Autodesk Fusion 360 part; units mm, degrees
(part 11 of 14)
  line L5327 (75.3115, 39.124) -> (75.7865, 39.124)
  line L5328 (77.3, 16.876) -> (76.5, 16.876)
  line L5329 (74.549, 38.8615) -> (74.549, 38.3865)
  line L5330 (75.3115, 40.124) -> (75.7865, 40.124)
  arc A2944 (81.0876, 38.2211) -> (81.0876, 38.4521) centre (81.0876, 38.3366) ccw
  line L5331 (75.049, 38.8615) -> (75.049, 38.3865)
  line L5332 (73.3115, 40.124) -> (73.7865, 40.124)
  arc A2945 (75.549, 38.6748) -> (75.549, 38.5732) centre (75.549, 38.624) ccw
  line L5333 (75.049, 40.8615) -> (75.049, 40.3865)
  line L5334 (75.3115, 39.624) -> (75.7865, 39.624)
  line L5335 (75.049, 38.8615) -> (75.049, 38.3865)
  arc A2946 (83.042, 40.8018) -> (83.042, 40.7002) centre (83.042, 40.751) ccw
  line L5336 (80.091, 16.622) -> (79.291, 16.622)
  line L5337 (73.3115, 39.124) -> (73.7865, 39.124)
  arc A2947 (75.549, 38.5732) -> (75.549, 38.6748) centre (75.549, 38.624) ccw
  line L5338 (75.549, 40.624) -> (73.549, 40.624)
  line L5339 (74.549, 40.174) -> (74.549, 39.074)
  line L5340 (74.049, 38.8615) -> (74.049, 38.3865)
  line L5341 (75.3115, 39.624) -> (75.7865, 39.624)
  line L5342 (74.549, 40.174) -> (74.549, 39.074)
  line L5343 (80.091, 17.272) -> (79.291, 17.272)
  line L5344 (73.549, 40.624) -> (73.549, 38.624)
  line L5345 (77.3, 16.876) -> (76.5, 16.876)
  line L5346 (80.091, 16.622) -> (79.291, 16.622)
  arc A2948 (75.5034, 40.9229) -> (75.5034, 41.1539) centre (75.5034, 41.0384) ccw
  line L5347 (74.049, 38.8615) -> (74.049, 38.3865)
  line L5348 (74.549, 40.8615) -> (74.549, 40.3865)
  line L5349 (73.3115, 40.124) -> (73.7865, 40.124)
  line L5350 (74.549, 40.174) -> (74.549, 39.074)
  line L5351 (75.049, 40.8615) -> (75.049, 40.3865)
  arc A2949 (75.549, 40.6748) -> (75.549, 40.5732) centre (75.549, 40.624) ccw
  line L5352 (74.049, 40.8615) -> (74.049, 40.3865)
  line L5353 (75.9, 17.526) -> (75.1, 17.526)
  line L5354 (74.549, 40.8615) -> (74.549, 40.3865)
  arc A2950 (73.549, 38.6748) -> (73.549, 38.5732) centre (73.549, 38.624) ccw
  line L5355 (75.9, 18.176) -> (75.1, 18.176)
  arc A2951 (77.559, 16.5214) -> (77.559, 16.1966) centre (77.559, 16.359) ccw
  arc A2952 (73.549, 40.5732) -> (73.549, 40.6748) centre (73.549, 40.624) ccw
  arc A2953 (73.549, 38.5732) -> (73.549, 38.6748) centre (73.549, 38.624) ccw
  line L5356 (74.549, 40.8615) -> (74.549, 40.3865)
  line L5357 (73.3115, 39.624) -> (73.7865, 39.624)
  line L5358 (73.3115, 39.624) -> (73.7865, 39.624)
  line L5359 (75.549, 38.624) -> (75.549, 40.624)
  line L5360 (74.049, 40.8615) -> (74.049, 40.3865)
  line L5361 (73.3115, 40.124) -> (73.7865, 40.124)
  line L5362 (73.3115, 39.124) -> (73.7865, 39.124)
  line L5363 (73.549, 38.624) -> (75.549, 38.624)
  line L5364 (75.3115, 39.124) -> (75.7865, 39.124)
  line L5365 (75.9, 16.876) -> (75.1, 16.876)
  line L5366 (73.3115, 39.624) -> (73.7865, 39.624)
  arc A2954 (75.549, 40.5732) -> (75.549, 40.6748) centre (75.549, 40.624) ccw
  line L5367 (75.3115, 39.124) -> (75.7865, 39.124)
  line L5368 (74.549, 38.8615) -> (74.549, 38.3865)
  line L5369 (74.049, 38.8615) -> (74.049, 38.3865)
  line L5370 (75.9, 16.876) -> (75.1, 16.876)
  line L5371 (75.049, 40.8615) -> (75.049, 40.3865)
  arc A2955 (9.1123, 16.129) -> (11.2078, 16.129) centre (10.16, 16.129) ccw
  arc A2956 (10.16, 16.9227) -> (10.16, 15.3352) centre (10.16, 16.129) ccw
  arc A2957 (12.2555, 16.129) -> (8.0645, 16.129) centre (10.16, 16.129) ccw
  arc A2958 (10.16, 15.3352) -> (10.16, 16.9227) centre (10.16, 16.129) ccw
  arc A2959 (7.8105, 16.129) -> (12.5095, 16.129) centre (10.16, 16.129) ccw
  line L5372 (8.6783, 17.6107) -> (8.4987, 17.7903)
  line L5373 (11.507, 17.476) -> (11.8213, 17.7903)
  arc A2960 (9.2075, 16.129) -> (11.1125, 16.129) centre (10.16, 16.129) ccw
  line L5374 (11.6417, 17.6107) -> (11.8213, 17.7903)
  line L5375 (10.414, 16.129) -> (9.906, 16.129)
  line L5376 (10.414, 16.129) -> (9.906, 16.129)
  arc A2961 (10.16, 16.9227) -> (10.16, 15.3352) centre (10.16, 16.129) ccw
  arc A2962 (10.16, 16.9227) -> (10.16, 15.3352) centre (10.16, 16.129) ccw
  arc A2963 (12.5095, 16.129) -> (7.8105, 16.129) centre (10.16, 16.129) ccw
  arc A2964 (11.1125, 16.129) -> (9.2075, 16.129) centre (10.16, 16.129) ccw
  line L5377 (8.6783, 17.6107) -> (8.4987, 17.7903)
  line L5378 (11.6417, 14.6473) -> (11.8213, 14.4677)
  line L5379 (11.6417, 14.6473) -> (11.8213, 14.4677)
  arc A2965 (10.16, 16.9227) -> (10.16, 15.3352) centre (10.16, 16.129) ccw
  line L5380 (10.16, 15.875) -> (10.16, 16.383)
  line L5381 (10.16, 15.875) -> (10.16, 16.383)
  line L5382 (6.35, 11.43) -> (6.35, 11.938)
  arc A2966 (11.2078, 16.129) -> (9.1123, 16.129) centre (10.16, 16.129) ccw
  line L5383 (6.35, 11.43) -> (6.35, 11.938)
  line L5384 (6.35, 11.43) -> (6.35, 11.938)
  line L5385 (6.604, 11.684) -> (6.096, 11.684)
  arc A2967 (10.16, 16.9227) -> (10.16, 15.3352) centre (10.16, 16.129) ccw
  line L5386 (11.6417, 17.6107) -> (11.8213, 17.7903)
  arc A2968 (8.0645, 16.129) -> (12.2555, 16.129) centre (10.16, 16.129) ccw
  arc A2969 (10.16, 15.3352) -> (10.16, 16.9227) centre (10.16, 16.129) ccw
  line L5387 (5.6061, 17.9251) -> (5.6959, 18.0149)
  line L5388 (10.414, 16.129) -> (9.906, 16.129)
  arc A2970 (8.0645, 16.129) -> (12.2555, 16.129) centre (10.16, 16.129) ccw
  arc A2971 (12.5095, 16.129) -> (7.8105, 16.129) centre (10.16, 16.129) ccw
  line L5389 (10.16, 15.875) -> (10.16, 16.383)
  arc A2972 (10.16, 15.3352) -> (10.16, 16.9227) centre (10.16, 16.129) ccw
  arc A2973 (12.5095, 16.129) -> (7.8105, 16.129) centre (10.16, 16.129) ccw
  arc A2974 (10.16, 16.9227) -> (10.16, 15.3352) centre (10.16, 16.129) ccw
  line L5390 (10.414, 16.129) -> (9.906, 16.129)
  line L5391 (10.414, 16.129) -> (9.906, 16.129)
  line L5392 (10.16, 15.875) -> (10.16, 16.383)
  arc A2975 (12.065, 16.129) -> (8.255, 16.129) centre (10.16, 16.129) ccw
  line L5393 (10.414, 16.129) -> (9.906, 16.129)
  line L5394 (11.507, 14.782) -> (11.8213, 14.4677)
  line L5395 (10.414, 16.129) -> (9.906, 16.129)
  arc A2976 (7.8105, 16.129) -> (12.5095, 16.129) centre (10.16, 16.129) ccw
  arc A2977 (12.2555, 16.129) -> (8.0645, 16.129) centre (10.16, 16.129) ccw
  line L5396 (10.16, 15.875) -> (10.16, 16.383)
  arc A2978 (10.16, 15.3352) -> (10.16, 16.9227) centre (10.16, 16.129) ccw
  arc A2979 (10.16, 15.3352) -> (10.16, 16.9227) centre (10.16, 16.129) ccw
  arc A2980 (9.1123, 16.129) -> (11.2078, 16.129) centre (10.16, 16.129) ccw
  line L5397 (10.16, 15.875) -> (10.16, 16.383)
  line L5398 (8.6783, 14.6473) -> (8.4987, 14.4677)
  arc A2981 (7.8105, 16.129) -> (12.5095, 16.129) centre (10.16, 16.129) ccw
  arc A2982 (10.16, 15.3352) -> (10.16, 16.9227) centre (10.16, 16.129) ccw
  line L5399 (10.16, 15.875) -> (10.16, 16.383)
  line L5400 (8.813, 14.782) -> (8.4987, 14.4677)
  line L5401 (10.16, 15.875) -> (10.16, 16.383)
  line L5402 (8.6783, 14.6473) -> (8.4987, 14.4677)
  arc A2983 (10.16, 16.9227) -> (10.16, 15.3352) centre (10.16, 16.129) ccw
  arc A2984 (11.2078, 16.129) -> (9.1123, 16.129) centre (10.16, 16.129) ccw
  line L5403 (8.813, 17.476) -> (8.4987, 17.7903)
  arc A2985 (8.255, 16.129) -> (12.065, 16.129) centre (10.16, 16.129) ccw
  arc A2986 (10.16, 15.3352) -> (10.16, 16.9227) centre (10.16, 16.129) ccw
  arc A2987 (8.255, 11.684) -> (4.445, 11.684) centre (6.35, 11.684) ccw
  line L5404 (63.5, 5.588) -> (64.77, 6.858)
  line L5405 (60.96, 5.588) -> (62.23, 5.588)
  line L5406 (62.23, 6.858) -> (60.96, 6.858)
  line L5407 (59.69, 6.858) -> (58.42, 6.858)
  arc A2988 (6.35, 10.8902) -> (6.35, 12.4777) centre (6.35, 11.684) ccw
  arc A2989 (6.35, 10.8902) -> (6.35, 12.4777) centre (6.35, 11.684) ccw
  arc A2990 (11.2078, 16.129) -> (9.1123, 16.129) centre (10.16, 16.129) ccw
  line L5408 (6.35, 11.43) -> (6.35, 11.938)
  arc A2991 (4.2545, 11.684) -> (8.4455, 11.684) centre (6.35, 11.684) ccw
  arc A2992 (6.35, 12.4777) -> (6.35, 10.8902) centre (6.35, 11.684) ccw
  line L5409 (5.003, 13.031) -> (4.6887, 13.3453)
  arc A2993 (6.35, 10.8902) -> (6.35, 12.4777) centre (6.35, 11.684) ccw
  arc A2994 (4.0005, 11.684) -> (8.6995, 11.684) centre (6.35, 11.684) ccw
  arc A2995 (7.3978, 11.684) -> (5.3023, 11.684) centre (6.35, 11.684) ccw
  arc A2996 (6.35, 10.8902) -> (6.35, 12.4777) centre (6.35, 11.684) ccw
  line L5410 (6.35, 11.43) -> (6.35, 11.938)
  arc A2997 (6.35, 12.4777) -> (6.35, 10.8902) centre (6.35, 11.684) ccw
  arc A2998 (6.35, 12.4777) -> (6.35, 10.8902) centre (6.35, 11.684) ccw
  line L5411 (4.8683, 10.2023) -> (4.6887, 10.0227)
  line L5412 (57.15, 5.588) -> (55.88, 6.858)
  arc A2999 (6.35, 10.8902) -> (6.35, 12.4777) centre (6.35, 11.684) ccw
  arc A3000 (11.2078, 16.129) -> (9.1123, 16.129) centre (10.16, 16.129) ccw
  line L5413 (6.604, 11.684) -> (6.096, 11.684)
  arc A3001 (9.1123, 16.129) -> (11.2078, 16.129) centre (10.16, 16.129) ccw
  line L5414 (53.34, 5.588) -> (54.61, 6.858)
  line L5415 (7.8317, 13.1657) -> (8.0113, 13.3453)
  line L5416 (64.77, 5.588) -> (64.77, 6.858)
  arc A3002 (6.35, 10.8902) -> (6.35, 12.4777) centre (6.35, 11.684) ccw
  line L5417 (62.23, 5.588) -> (62.23, 6.858)
  line L5418 (7.8317, 10.2023) -> (8.0113, 10.0227)
  line L5419 (6.35, 11.43) -> (6.35, 11.938)
  line L5420 (55.88, 5.588) -> (57.15, 6.858)
  arc A3003 (5.3023, 11.684) -> (7.3978, 11.684) centre (6.35, 11.684) ccw
  line L5421 (52.705, 7.493) -> (52.705, 2.413)
  arc A3004 (6.35, 12.4777) -> (6.35, 10.8902) centre (6.35, 11.684) ccw
  line L5422 (6.604, 11.684) -> (6.096, 11.684)
  line L5423 (6.35, 11.43) -> (6.35, 11.938)
  arc A3005 (5.3023, 11.684) -> (7.3978, 11.684) centre (6.35, 11.684) ccw
  arc A3006 (6.35, 12.4777) -> (6.35, 10.8902) centre (6.35, 11.684) ccw
  arc A3007 (6.35, 10.8902) -> (6.35, 12.4777) centre (6.35, 11.684) ccw
  arc A3008 (6.35, 12.4777) -> (6.35, 10.8902) centre (6.35, 11.684) ccw
  arc A3009 (6.35, 12.4777) -> (6.35, 10.8902) centre (6.35, 11.684) ccw
  line L5424 (6.35, 11.43) -> (6.35, 11.938)
  line L5425 (6.604, 11.684) -> (6.096, 11.684)
  line L5426 (6.604, 11.684) -> (6.096, 11.684)
  line L5427 (6.604, 11.684) -> (6.096, 11.684)
  line L5428 (6.35, 11.43) -> (6.35, 11.938)
  line L5429 (6.604, 11.684) -> (6.096, 11.684)
  line L5430 (6.604, 11.684) -> (6.096, 11.684)
  arc A3010 (6.35, 12.4777) -> (6.35, 10.8902) centre (6.35, 11.684) ccw
  line L5431 (6.604, 11.684) -> (6.096, 11.684)
  line L5432 (6.604, 11.684) -> (6.096, 11.684)
  line L5433 (6.35, 11.43) -> (6.35, 11.938)
  arc A3011 (6.35, 10.8902) -> (6.35, 12.4777) centre (6.35, 11.684) ccw
  arc A3012 (6.35, 12.4777) -> (6.35, 10.8902) centre (6.35, 11.684) ccw
  arc A3013 (6.35, 10.8902) -> (6.35, 12.4777) centre (6.35, 11.684) ccw
  arc A3014 (6.35, 12.4777) -> (6.35, 10.8902) centre (6.35, 11.684) ccw
  arc A3015 (8.4455, 11.684) -> (4.2545, 11.684) centre (6.35, 11.684) ccw
  arc A3016 (4.2545, 11.684) -> (8.4455, 11.684) centre (6.35, 11.684) ccw
  line L5434 (7.8317, 10.2023) -> (8.0113, 10.0227)
  arc A3017 (9.1123, 16.129) -> (11.2078, 16.129) centre (10.16, 16.129) ccw
  line L5435 (4.8683, 13.1657) -> (4.6887, 13.3453)
  arc A3018 (6.35, 10.8902) -> (6.35, 12.4777) centre (6.35, 11.684) ccw
  line L5436 (54.61, 5.588) -> (54.61, 6.858)
  line L5437 (65.405, 7.493) -> (52.705, 7.493)
  arc A3019 (5.3023, 11.684) -> (7.3978, 11.684) centre (6.35, 11.684) ccw
  line L5438 (4.8683, 13.1657) -> (4.6887, 13.3453)
  line L5439 (64.77, 6.858) -> (63.5, 6.858)
  line L5440 (55.88, 6.858) -> (55.88, 5.588)
  line L5441 (58.42, 3.048) -> (59.69, 3.048)
  line L5442 (60.96, 6.858) -> (60.96, 5.588)
  arc A3020 (8.4455, 11.684) -> (4.2545, 11.684) centre (6.35, 11.684) ccw
  line L5443 (64.77, 3.048) -> (64.77, 4.318)
  line L5444 (58.42, 4.318) -> (58.42, 3.048)
  arc A3021 (4.0005, 11.684) -> (8.6995, 11.684) centre (6.35, 11.684) ccw
  line L5445 (58.42, 5.588) -> (59.69, 6.858)
  arc A3022 (8.6995, 11.684) -> (4.0005, 11.684) centre (6.35, 11.684) ccw
  arc A3023 (7.3025, 11.684) -> (5.3975, 11.684) centre (6.35, 11.684) ccw
  line L5446 (63.5, 6.858) -> (63.5, 5.588)
  line L5447 (55.88, 3.048) -> (57.15, 3.048)
  line L5448 (53.975, 3.937) -> (53.975, 3.429)
  line L5449 (60.325, 2.413) -> (60.325, 7.493)
  line L5450 (57.15, 6.858) -> (55.88, 6.858)
  line L5451 (52.705, 2.413) -> (65.405, 2.413)
  line L5452 (55.88, 5.588) -> (57.15, 5.588)
  line L5453 (52.705, 7.493) -> (52.705, 2.413)
  line L5454 (64.77, 4.318) -> (63.5, 4.318)
  line L5455 (60.96, 4.318) -> (60.96, 3.048)
  line L5456 (57.15, 4.318) -> (55.88, 4.318)
  line L5457 (7.697, 10.337) -> (8.0113, 10.0227)
  line L5458 (58.42, 3.048) -> (59.69, 4.318)
  line L5459 (59.69, 3.048) -> (59.69, 4.318)
  line L5460 (62.23, 5.588) -> (60.96, 6.858)
  arc A3024 (5.3975, 11.684) -> (7.3025, 11.684) centre (6.35, 11.684) ccw
  arc A3025 (7.3978, 11.684) -> (5.3023, 11.684) centre (6.35, 11.684) ccw
  line L5461 (59.69, 5.588) -> (58.42, 6.858)
  line L5462 (60.96, 5.588) -> (62.23, 6.858)
  line L5463 (5.003, 10.337) -> (4.6887, 10.0227)
  line L5464 (54.61, 4.318) -> (53.34, 4.318)
  line L5465 (58.42, 6.858) -> (58.42, 5.588)
  arc A3026 (7.3978, 11.684) -> (5.3023, 11.684) centre (6.35, 11.684) ccw
  arc A3027 (8.6995, 11.684) -> (4.0005, 11.684) centre (6.35, 11.684) ccw
  line L5466 (7.697, 13.031) -> (8.0113, 13.3453)
  arc A3028 (5.3023, 11.684) -> (7.3978, 11.684) centre (6.35, 11.684) ccw
  line L5467 (62.23, 3.048) -> (62.23, 4.318)
  line L5468 (59.69, 5.588) -> (59.69, 6.858)
  line L5469 (63.5, 5.588) -> (64.77, 5.588)
  line L5470 (59.69, 3.048) -> (58.42, 4.318)
  line L5471 (62.23, 3.048) -> (60.96, 4.318)
  line L5472 (60.96, 3.048) -> (62.23, 4.318)
  line L5473 (53.34, 5.588) -> (54.61, 5.588)
  line L5474 (57.785, 2.413) -> (57.785, 7.493)
  line L5475 (54.61, 5.588) -> (53.34, 6.858)
  line L5476 (65.405, 7.493) -> (52.705, 7.493)
  arc A3029 (7.3978, 11.684) -> (5.3023, 11.684) centre (6.35, 11.684) ccw
  line L5477 (62.865, 2.413) -> (62.865, 7.493)
  line L5478 (53.34, 3.048) -> (54.61, 3.048)
  line L5479 (64.77, 5.588) -> (63.5, 6.858)
  line L5480 (65.405, 2.413) -> (65.405, 7.493)
  arc A3030 (54.2227, 3.683) -> (53.7274, 3.683) centre (53.975, 3.683) ccw
  arc A3031 (4.445, 11.684) -> (8.255, 11.684) centre (6.35, 11.684) ccw
  line L5481 (52.705, 2.413) -> (65.405, 2.413)
  line L5482 (55.88, 3.048) -> (57.15, 4.318)
  line L5483 (54.61, 3.048) -> (53.34, 4.318)
  line L5484 (55.88, 4.318) -> (55.88, 3.048)
  line L5485 (62.23, 4.318) -> (60.96, 4.318)
  line L5486 (57.15, 3.048) -> (55.88, 4.318)
  line L5487 (53.975, 6.477) -> (53.975, 5.969)
  arc A3032 (54.2227, 3.683) -> (53.7274, 3.683) centre (53.975, 3.683) ccw
  line L5488 (54.229, 3.683) -> (53.721, 3.683)
  arc A3033 (53.7274, 3.683) -> (54.2227, 3.683) centre (53.975, 3.683) ccw
  line L5489 (53.975, 3.937) -> (53.975, 3.429)
  line L5490 (63.5, 3.048) -> (64.77, 4.318)
  line L5491 (57.15, 5.588) -> (57.15, 6.858)
  line L5492 (53.34, 3.048) -> (54.61, 4.318)
  line L5493 (54.229, 3.683) -> (53.721, 3.683)
  line L5494 (58.42, 5.588) -> (59.69, 5.588)
  line L5495 (53.975, 6.477) -> (53.975, 5.969)
  line L5496 (54.7624, 3.683) -> (53.1876, 3.683)
  arc A3034 (53.7274, 3.683) -> (54.2227, 3.683) centre (53.975, 3.683) ccw
  line L5497 (54.229, 6.223) -> (53.721, 6.223)
  arc A3035 (53.7274, 3.683) -> (54.2227, 3.683) centre (53.975, 3.683) ccw
  line L5498 (54.7624, 3.683) -> (53.1876, 3.683)
  line L5499 (63.5, 3.048) -> (64.77, 3.048)
  arc A3036 (53.7274, 3.683) -> (54.2227, 3.683) centre (53.975, 3.683) ccw
  line L5500 (54.229, 6.223) -> (53.721, 6.223)
  arc A3037 (54.2227, 3.683) -> (53.7274, 3.683) centre (53.975, 3.683) ccw
  line L5501 (54.61, 3.048) -> (54.61, 4.318)
  line L5502 (57.15, 3.048) -> (57.15, 4.318)
  arc A3038 (53.975, 3.429) -> (53.975, 3.937) centre (53.975, 3.683) ccw
  line L5503 (53.975, 6.477) -> (53.975, 5.969)
  line L5504 (54.229, 3.683) -> (53.721, 3.683)
  line L5505 (53.975, 6.477) -> (53.975, 5.969)
  arc A3039 (53.7274, 3.683) -> (54.2227, 3.683) centre (53.975, 3.683) ccw
  arc A3040 (54.2227, 6.223) -> (53.7274, 6.223) centre (53.975, 6.223) ccw
  line L5506 (64.77, 3.048) -> (63.5, 4.318)
  line L5507 (54.7624, 3.683) -> (53.1876, 3.683)
  line L5508 (53.34, 4.318) -> (53.34, 3.048)
  arc A3041 (54.2227, 3.683) -> (53.7274, 3.683) centre (53.975, 3.683) ccw
  arc A3042 (54.2227, 3.683) -> (53.7274, 3.683) centre (53.975, 3.683) ccw
  arc A3043 (53.7274, 3.683) -> (54.2227, 3.683) centre (53.975, 3.683) ccw
  line L5509 (63.5, 4.318) -> (63.5, 3.048)
  line L5510 (54.229, 3.683) -> (53.721, 3.683)
  arc A3044 (54.2227, 6.223) -> (53.7274, 6.223) centre (53.975, 6.223) ccw
  arc A3045 (53.7274, 3.683) -> (54.2227, 3.683) centre (53.975, 3.683) ccw
  line L5511 (59.69, 4.318) -> (58.42, 4.318)
  line L5512 (54.229, 3.683) -> (53.721, 3.683)
  line L5513 (53.975, 3.937) -> (53.975, 3.429)
  arc A3046 (54.2227, 6.223) -> (53.7274, 6.223) centre (53.975, 6.223) ccw
  line L5514 (54.7624, 3.683) -> (53.1876, 3.683)
  arc A3047 (53.7274, 3.683) -> (54.2227, 3.683) centre (53.975, 3.683) ccw
  line L5515 (54.229, 3.683) -> (53.721, 3.683)
  arc A3048 (53.975, 4.0767) -> (53.975, 3.2893) centre (53.975, 3.683) ccw
  line L5516 (55.245, 2.413) -> (55.245, 7.493)
  line L5517 (53.34, 6.858) -> (53.34, 5.588)
  arc A3049 (53.975, 3.937) -> (53.975, 3.429) centre (53.975, 3.683) ccw
  line L5518 (53.975, 3.937) -> (53.975, 3.429)
  line L5519 (60.96, 3.048) -> (62.23, 3.048)
  line L5520 (65.405, 2.413) -> (65.405, 7.493)
  arc A3050 (54.2227, 3.683) -> (53.7274, 3.683) centre (53.975, 3.683) ccw
  arc A3051 (53.7274, 3.683) -> (54.2227, 3.683) centre (53.975, 3.683) ccw
  line L5521 (54.229, 3.683) -> (53.721, 3.683)
  arc A3052 (54.2227, 3.683) -> (53.7274, 3.683) centre (53.975, 3.683) ccw
  line L5522 (54.61, 6.858) -> (53.34, 6.858)
  line L5523 (53.975, 3.937) -> (53.975, 3.429)
  line L5524 (53.975, 3.937) -> (53.975, 3.429)
  arc A3053 (53.975, 3.2893) -> (53.975, 4.0767) centre (53.975, 3.683) ccw
  line L5525 (54.229, 6.223) -> (53.721, 6.223)
  arc A3054 (53.7274, 6.223) -> (54.2227, 6.223) centre (53.975, 6.223) ccw
  arc A3055 (54.2227, 3.683) -> (53.7274, 3.683) centre (53.975, 3.683) ccw
  line L5526 (54.229, 3.683) -> (53.721, 3.683)
  arc A3056 (56.7627, 3.683) -> (56.2674, 3.683) centre (56.515, 3.683) ccw
  line L5527 (53.975, 6.477) -> (53.975, 5.969)
  line L5528 (53.975, 3.937) -> (53.975, 3.429)
  line L5529 (53.975, 3.937) -> (53.975, 3.429)
  arc A3057 (56.2674, 3.683) -> (56.7627, 3.683) centre (56.515, 3.683) ccw
  arc A3058 (54.2227, 6.223) -> (53.7274, 6.223) centre (53.975, 6.223) ccw
  arc A3059 (56.2674, 3.683) -> (56.7627, 3.683) centre (56.515, 3.683) ccw
  line L5530 (54.229, 6.223) -> (53.721, 6.223)
  line L5531 (53.975, 6.477) -> (53.975, 5.969)
  line L5532 (53.975, 3.937) -> (53.975, 3.429)
  line L5533 (54.229, 6.223) -> (53.721, 6.223)
  arc A3060 (56.2674, 3.683) -> (56.7627, 3.683) centre (56.515, 3.683) ccw
  arc A3061 (56.2674, 3.683) -> (56.7627, 3.683) centre (56.515, 3.683) ccw
  arc A3062 (56.7627, 3.683) -> (56.2674, 3.683) centre (56.515, 3.683) ccw
  arc A3063 (56.2674, 3.683) -> (56.7627, 3.683) centre (56.515, 3.683) ccw
  line L5534 (56.515, 3.937) -> (56.515, 3.429)
  arc A3064 (53.7274, 6.223) -> (54.2227, 6.223) centre (53.975, 6.223) ccw
  arc A3065 (54.2227, 3.683) -> (53.7274, 3.683) centre (53.975, 3.683) ccw
  line L5535 (56.515, 3.937) -> (56.515, 3.429)
  arc A3066 (53.975, 6.477) -> (53.975, 5.969) centre (53.975, 6.223) ccw
  arc A3067 (54.2227, 6.223) -> (53.7274, 6.223) centre (53.975, 6.223) ccw
  arc A3068 (53.7274, 6.223) -> (54.2227, 6.223) centre (53.975, 6.223) ccw
  arc A3069 (54.2227, 6.223) -> (53.7274, 6.223) centre (53.975, 6.223) ccw
  line L5536 (56.515, 3.937) -> (56.515, 3.429)
  line L5537 (56.769, 3.683) -> (56.261, 3.683)
  arc A3070 (53.975, 6.6167) -> (53.975, 5.8293) centre (53.975, 6.223) ccw
  arc A3071 (56.7627, 3.683) -> (56.2674, 3.683) centre (56.515, 3.683) ccw
  arc A3072 (53.975, 6.6167) -> (53.975, 5.8293) centre (53.975, 6.223) ccw
  arc A3073 (53.7274, 3.683) -> (54.2227, 3.683) centre (53.975, 3.683) ccw
  line L5538 (54.229, 6.223) -> (53.721, 6.223)
  arc A3074 (54.2227, 3.683) -> (53.7274, 3.683) centre (53.975, 3.683) ccw
  arc A3075 (53.7274, 6.223) -> (54.2227, 6.223) centre (53.975, 6.223) ccw
  line L5539 (56.769, 3.683) -> (56.261, 3.683)
  line L5540 (53.975, 6.477) -> (53.975, 5.969)
  arc A3076 (56.2674, 3.683) -> (56.7627, 3.683) centre (56.515, 3.683) ccw
  arc A3077 (53.975, 6.6167) -> (53.975, 5.8293) centre (53.975, 6.223) ccw
  line L5541 (56.515, 3.937) -> (56.515, 3.429)
  arc A3078 (56.7627, 3.683) -> (56.2674, 3.683) centre (56.515, 3.683) ccw
  line L5542 (54.229, 6.223) -> (53.721, 6.223)
  line L5543 (53.975, 6.477) -> (53.975, 5.969)
  line L5544 (54.229, 6.223) -> (53.721, 6.223)
  line L5545 (53.975, 3.937) -> (53.975, 3.429)
  arc A3079 (53.975, 6.6167) -> (53.975, 5.8293) centre (53.975, 6.223) ccw
  arc A3080 (54.2227, 6.223) -> (53.7274, 6.223) centre (53.975, 6.223) ccw
  line L5546 (54.229, 3.683) -> (53.721, 3.683)
  line L5547 (56.515, 3.937) -> (56.515, 3.429)
  arc A3081 (56.7627, 3.683) -> (56.2674, 3.683) centre (56.515, 3.683) ccw
  line L5548 (54.229, 3.683) -> (53.721, 3.683)
  line L5549 (53.975, 6.477) -> (53.975, 5.969)
  line L5550 (56.769, 3.683) -> (56.261, 3.683)
  arc A3082 (54.2227, 6.223) -> (53.7274, 6.223) centre (53.975, 6.223) ccw
  arc A3083 (56.7627, 3.683) -> (56.2674, 3.683) centre (56.515, 3.683) ccw
  arc A3084 (53.7274, 6.223) -> (54.2227, 6.223) centre (53.975, 6.223) ccw
  line L5551 (56.515, 3.937) -> (56.515, 3.429)
  line L5552 (54.229, 6.223) -> (53.721, 6.223)
  arc A3085 (53.7274, 6.223) -> (54.2227, 6.223) centre (53.975, 6.223) ccw
  arc A3086 (53.7274, 6.223) -> (54.2227, 6.223) centre (53.975, 6.223) ccw
  arc A3087 (54.2227, 6.223) -> (53.7274, 6.223) centre (53.975, 6.223) ccw
  line L5553 (53.975, 6.477) -> (53.975, 5.969)
  arc A3088 (53.975, 5.969) -> (53.975, 6.477) centre (53.975, 6.223) ccw
  line L5554 (56.769, 3.683) -> (56.261, 3.683)
  arc A3089 (53.975, 6.6167) -> (53.975, 5.8293) centre (53.975, 6.223) ccw
  arc A3090 (53.7274, 6.223) -> (54.2227, 6.223) centre (53.975, 6.223) ccw
  arc A3091 (53.975, 5.8293) -> (53.975, 6.6167) centre (53.975, 6.223) ccw
  arc A3092 (56.7627, 3.683) -> (56.2674, 3.683) centre (56.515, 3.683) ccw
  arc A3093 (56.515, 3.2893) -> (56.515, 4.0767) centre (56.515, 3.683) ccw
  line L5555 (54.229, 6.223) -> (53.721, 6.223)
  arc A3094 (56.515, 3.2893) -> (56.515, 4.0767) centre (56.515, 3.683) ccw
  arc A3095 (56.515, 3.2893) -> (56.515, 4.0767) centre (56.515, 3.683) ccw
  line L5556 (56.515, 6.477) -> (56.515, 5.969)
  arc A3096 (56.7627, 6.223) -> (56.2674, 6.223) centre (56.515, 6.223) ccw
  arc A3097 (53.975, 5.8293) -> (53.975, 6.6167) centre (53.975, 6.223) ccw
  arc A3098 (56.515, 4.0767) -> (56.515, 3.2893) centre (56.515, 3.683) ccw
  arc A3099 (56.2674, 6.223) -> (56.7627, 6.223) centre (56.515, 6.223) ccw
  line L5557 (56.515, 6.477) -> (56.515, 5.969)
  arc A3100 (54.2227, 6.223) -> (53.7274, 6.223) centre (53.975, 6.223) ccw
  line L5558 (56.769, 3.683) -> (56.261, 3.683)
  arc A3101 (56.7627, 3.683) -> (56.2674, 3.683) centre (56.515, 3.683) ccw
  line L5559 (56.769, 6.223) -> (56.261, 6.223)
  arc A3102 (56.515, 3.937) -> (56.515, 3.429) centre (56.515, 3.683) ccw
  line L5560 (56.769, 3.683) -> (56.261, 3.683)
  arc A3103 (56.2674, 3.683) -> (56.7627, 3.683) centre (56.515, 3.683) ccw
  arc A3104 (56.7627, 6.223) -> (56.2674, 6.223) centre (56.515, 6.223) ccw
  arc A3105 (53.975, 5.8293) -> (53.975, 6.6167) centre (53.975, 6.223) ccw
  arc A3106 (56.7627, 6.223) -> (56.2674, 6.223) centre (56.515, 6.223) ccw
  line L5561 (56.515, 6.477) -> (56.515, 5.969)
  line L5562 (56.769, 3.683) -> (56.261, 3.683)
  line L5563 (56.769, 6.223) -> (56.261, 6.223)
  line L5564 (56.769, 6.223) -> (56.261, 6.223)
  arc A3107 (56.2674, 6.223) -> (56.7627, 6.223) centre (56.515, 6.223) ccw
  line L5565 (56.769, 6.223) -> (56.261, 6.223)
  arc A3108 (56.2674, 6.223) -> (56.7627, 6.223) centre (56.515, 6.223) ccw
  line L5566 (56.515, 6.477) -> (56.515, 5.969)
  arc A3109 (56.515, 4.0767) -> (56.515, 3.2893) centre (56.515, 3.683) ccw
  line L5567 (56.515, 6.477) -> (56.515, 5.969)
  arc A3110 (56.2674, 6.223) -> (56.7627, 6.223) centre (56.515, 6.223) ccw
  arc A3111 (56.7627, 3.683) -> (56.2674, 3.683) centre (56.515, 3.683) ccw
  arc A3112 (56.2674, 6.223) -> (56.7627, 6.223) centre (56.515, 6.223) ccw
  arc A3113 (56.2674, 3.683) -> (56.7627, 3.683) centre (56.515, 3.683) ccw
  line L5568 (56.515, 3.937) -> (56.515, 3.429)
  arc A3114 (56.7627, 6.223) -> (56.2674, 6.223) centre (56.515, 6.223) ccw
  line L5569 (56.769, 6.223) -> (56.261, 6.223)
  arc A3115 (56.7627, 6.223) -> (56.2674, 6.223) centre (56.515, 6.223) ccw
  line L5570 (56.769, 6.223) -> (56.261, 6.223)
  arc A3116 (56.7627, 3.683) -> (56.2674, 3.683) centre (56.515, 3.683) ccw
  line L5571 (56.515, 6.477) -> (56.515, 5.969)
  arc A3117 (56.7627, 6.223) -> (56.2674, 6.223) centre (56.515, 6.223) ccw
  arc A3118 (56.515, 4.0767) -> (56.515, 3.2893) centre (56.515, 3.683) ccw
  arc A3119 (56.515, 3.2893) -> (56.515, 4.0767) centre (56.515, 3.683) ccw
  arc A3120 (56.7627, 6.223) -> (56.2674, 6.223) centre (56.515, 6.223) ccw
  arc A3121 (53.7274, 6.223) -> (54.2227, 6.223) centre (53.975, 6.223) ccw
  arc A3122 (53.975, 5.8293) -> (53.975, 6.6167) centre (53.975, 6.223) ccw
  arc A3123 (56.515, 4.0767) -> (56.515, 3.2893) centre (56.515, 3.683) ccw
  line L5572 (56.515, 6.477) -> (56.515, 5.969)
  line L5573 (56.769, 6.223) -> (56.261, 6.223)
  arc A3124 (56.2674, 3.683) -> (56.7627, 3.683) centre (56.515, 3.683) ccw
  line L5574 (56.769, 3.683) -> (56.261, 3.683)
  arc A3125 (53.975, 5.8293) -> (53.975, 6.6167) centre (53.975, 6.223) ccw
  arc A3126 (53.7274, 6.223) -> (54.2227, 6.223) centre (53.975, 6.223) ccw
  arc A3127 (56.515, 3.429) -> (56.515, 3.937) centre (56.515, 3.683) ccw
  line L5575 (56.515, 3.937) -> (56.515, 3.429)
  arc A3128 (56.2674, 6.223) -> (56.7627, 6.223) centre (56.515, 6.223) ccw
  arc A3129 (56.7627, 6.223) -> (56.2674, 6.223) centre (56.515, 6.223) ccw
  line L5576 (56.515, 6.477) -> (56.515, 5.969)
  line L5577 (56.769, 3.683) -> (56.261, 3.683)
  arc A3130 (56.2674, 3.683) -> (56.7627, 3.683) centre (56.515, 3.683) ccw
  arc A3131 (56.7627, 6.223) -> (56.2674, 6.223) centre (56.515, 6.223) ccw
  line L5578 (56.515, 3.937) -> (56.515, 3.429)
  arc A3132 (56.2674, 6.223) -> (56.7627, 6.223) centre (56.515, 6.223) ccw
  arc A3133 (58.8073, 3.683) -> (59.3027, 3.683) centre (59.055, 3.683) ccw
  line L5579 (59.309, 3.683) -> (58.801, 3.683)
  line L5580 (59.309, 3.683) -> (58.801, 3.683)
  line L5581 (59.055, 3.937) -> (59.055, 3.429)
  line L5582 (59.055, 3.937) -> (59.055, 3.429)
  line L5583 (59.055, 3.937) -> (59.055, 3.429)
  arc A3134 (56.515, 6.6167) -> (56.515, 5.8293) centre (56.515, 6.223) ccw
  arc A3135 (58.8073, 3.683) -> (59.3027, 3.683) centre (59.055, 3.683) ccw
  arc A3136 (59.3027, 3.683) -> (58.8073, 3.683) centre (59.055, 3.683) ccw
  arc A3137 (58.8073, 3.683) -> (59.3027, 3.683) centre (59.055, 3.683) ccw
  arc A3138 (58.8073, 3.683) -> (59.3027, 3.683) centre (59.055, 3.683) ccw
  line L5584 (56.515, 6.477) -> (56.515, 5.969)
  line L5585 (59.309, 3.683) -> (58.801, 3.683)
  arc A3139 (56.515, 5.969) -> (56.515, 6.477) centre (56.515, 6.223) ccw
  line L5586 (59.055, 3.937) -> (59.055, 3.429)
  line L5587 (59.055, 3.937) -> (59.055, 3.429)
  arc A3140 (58.8073, 3.683) -> (59.3027, 3.683) centre (59.055, 3.683) ccw
  arc A3141 (56.2674, 6.223) -> (56.7627, 6.223) centre (56.515, 6.223) ccw
  line L5588 (59.309, 3.683) -> (58.801, 3.683)
  arc A3142 (58.8073, 3.683) -> (59.3027, 3.683) centre (59.055, 3.683) ccw
  line L5589 (56.769, 3.683) -> (56.261, 3.683)
  arc A3143 (56.515, 5.8293) -> (56.515, 6.6167) centre (56.515, 6.223) ccw
  line L5590 (56.515, 6.477) -> (56.515, 5.969)
  line L5591 (59.309, 3.683) -> (58.801, 3.683)
  line L5592 (56.769, 6.223) -> (56.261, 6.223)
  arc A3144 (56.515, 6.6167) -> (56.515, 5.8293) centre (56.515, 6.223) ccw
  arc A3145 (59.3027, 3.683) -> (58.8073, 3.683) centre (59.055, 3.683) ccw
  arc A3146 (58.8073, 3.683) -> (59.3027, 3.683) centre (59.055, 3.683) ccw
  arc A3147 (56.515, 6.6167) -> (56.515, 5.8293) centre (56.515, 6.223) ccw
  line L5593 (59.055, 3.937) -> (59.055, 3.429)
  arc A3148 (59.3027, 3.683) -> (58.8073, 3.683) centre (59.055, 3.683) ccw
  line L5594 (59.055, 3.937) -> (59.055, 3.429)
  arc A3149 (58.8073, 3.683) -> (59.3027, 3.683) centre (59.055, 3.683) ccw
  arc A3150 (56.515, 6.6167) -> (56.515, 5.8293) centre (56.515, 6.223) ccw
  arc A3151 (56.7627, 6.223) -> (56.2674, 6.223) centre (56.515, 6.223) ccw
  arc A3152 (59.3027, 3.683) -> (58.8073, 3.683) centre (59.055, 3.683) ccw
  arc A3153 (56.515, 5.8293) -> (56.515, 6.6167) centre (56.515, 6.223) ccw
  arc A3154 (59.3027, 3.683) -> (58.8073, 3.683) centre (59.055, 3.683) ccw
  arc A3155 (56.515, 6.6167) -> (56.515, 5.8293) centre (56.515, 6.223) ccw
  arc A3156 (56.515, 4.0767) -> (56.515, 3.2893) centre (56.515, 3.683) ccw
  arc A3157 (59.3027, 3.683) -> (58.8073, 3.683) centre (59.055, 3.683) ccw
  arc A3158 (58.8073, 3.683) -> (59.3027, 3.683) centre (59.055, 3.683) ccw
  line L5595 (59.309, 3.683) -> (58.801, 3.683)
  line L5596 (59.055, 3.937) -> (59.055, 3.429)
  arc A3159 (56.515, 5.8293) -> (56.515, 6.6167) centre (56.515, 6.223) ccw
  arc A3160 (59.3027, 3.683) -> (58.8073, 3.683) centre (59.055, 3.683) ccw
  arc A3161 (56.515, 6.477) -> (56.515, 5.969) centre (56.515, 6.223) ccw
  arc A3162 (58.8073, 3.683) -> (59.3027, 3.683) centre (59.055, 3.683) ccw
  line L5597 (59.309, 3.683) -> (58.801, 3.683)
  arc A3163 (56.515, 3.2893) -> (56.515, 4.0767) centre (56.515, 3.683) ccw
  arc A3164 (56.515, 5.8293) -> (56.515, 6.6167) centre (56.515, 6.223) ccw
  line L5598 (56.515, 3.937) -> (56.515, 3.429)
  line L5599 (56.769, 6.223) -> (56.261, 6.223)
  arc A3165 (56.2674, 6.223) -> (56.7627, 6.223) centre (56.515, 6.223) ccw
  arc A3166 (56.515, 5.8293) -> (56.515, 6.6167) centre (56.515, 6.223) ccw
  arc A3167 (59.3027, 3.683) -> (58.8073, 3.683) centre (59.055, 3.683) ccw
  arc A3168 (59.3027, 3.683) -> (58.8073, 3.683) centre (59.055, 3.683) ccw
  arc A3169 (59.3027, 3.683) -> (58.8073, 3.683) centre (59.055, 3.683) ccw
  line L5600 (56.769, 6.223) -> (56.261, 6.223)
  line L5601 (59.309, 3.683) -> (58.801, 3.683)
  line L5602 (59.309, 3.683) -> (58.801, 3.683)
  arc A3170 (56.2674, 6.223) -> (56.7627, 6.223) centre (56.515, 6.223) ccw
  line L5603 (59.055, 3.937) -> (59.055, 3.429)
  line L5604 (59.055, 6.477) -> (59.055, 5.969)
  line L5605 (59.309, 6.223) -> (58.801, 6.223)
  arc A3171 (58.8073, 6.223) -> (59.3027, 6.223) centre (59.055, 6.223) ccw
  arc A3172 (59.3027, 6.223) -> (58.8073, 6.223) centre (59.055, 6.223) ccw
  arc A3173 (59.055, 4.0767) -> (59.055, 3.2893) centre (59.055, 3.683) ccw
  arc A3174 (59.055, 4.0767) -> (59.055, 3.2893) centre (59.055, 3.683) ccw
  line L5606 (59.055, 6.477) -> (59.055, 5.969)
  arc A3175 (58.8073, 6.223) -> (59.3027, 6.223) centre (59.055, 6.223) ccw
  line L5607 (61.595, 3.937) -> (61.595, 3.429)
  arc A3176 (61.8427, 3.683) -> (61.3473, 3.683) centre (61.595, 3.683) ccw
  arc A3177 (59.3027, 6.223) -> (58.8073, 6.223) centre (59.055, 6.223) ccw
  arc A3178 (59.3027, 6.223) -> (58.8073, 6.223) centre (59.055, 6.223) ccw
  arc A3179 (59.055, 3.937) -> (59.055, 3.429) centre (59.055, 3.683) ccw
  arc A3180 (61.8427, 3.683) -> (61.3473, 3.683) centre (61.595, 3.683) ccw
  line L5608 (59.309, 6.223) -> (58.801, 6.223)
  arc A3181 (59.3027, 6.223) -> (58.8073, 6.223) centre (59.055, 6.223) ccw
  arc A3182 (58.8073, 6.223) -> (59.3027, 6.223) centre (59.055, 6.223) ccw
  arc A3183 (61.595, 4.0767) -> (61.595, 3.2893) centre (61.595, 3.683) ccw
  arc A3184 (58.8073, 6.223) -> (59.3027, 6.223) centre (59.055, 6.223) ccw
  line L5609 (59.055, 6.477) -> (59.055, 5.969)
  line L5610 (59.309, 6.223) -> (58.801, 6.223)
  arc A3185 (59.055, 3.2893) -> (59.055, 4.0767) centre (59.055, 3.683) ccw
  line L5611 (59.055, 6.477) -> (59.055, 5.969)
  line L5612 (59.055, 6.477) -> (59.055, 5.969)
  line L5613 (59.309, 6.223) -> (58.801, 6.223)
  line L5614 (59.309, 6.223) -> (58.801, 6.223)
  line L5615 (59.309, 6.223) -> (58.801, 6.223)
  arc A3186 (59.3027, 6.223) -> (58.8073, 6.223) centre (59.055, 6.223) ccw
  line L5616 (61.849, 3.683) -> (61.341, 3.683)
  arc A3187 (58.8073, 6.223) -> (59.3027, 6.223) centre (59.055, 6.223) ccw
  arc A3188 (59.055, 3.2893) -> (59.055, 4.0767) centre (59.055, 3.683) ccw
  arc A3189 (58.8073, 6.223) -> (59.3027, 6.223) centre (59.055, 6.223) ccw
  arc A3190 (59.3027, 6.223) -> (58.8073, 6.223) centre (59.055, 6.223) ccw
  arc A3191 (59.055, 3.2893) -> (59.055, 4.0767) centre (59.055, 3.683) ccw
  arc A3192 (59.3027, 6.223) -> (58.8073, 6.223) centre (59.055, 6.223) ccw
  line L5617 (61.595, 3.937) -> (61.595, 3.429)
  arc A3193 (61.8427, 3.683) -> (61.3473, 3.683) centre (61.595, 3.683) ccw
  arc A3194 (59.055, 3.429) -> (59.055, 3.937) centre (59.055, 3.683) ccw
  arc A3195 (59.055, 4.0767) -> (59.055, 3.2893) centre (59.055, 3.683) ccw
  line L5618 (61.595, 3.937) -> (61.595, 3.429)
  line L5619 (59.055, 6.477) -> (59.055, 5.969)
  arc A3196 (58.8073, 6.223) -> (59.3027, 6.223) centre (59.055, 6.223) ccw
  line L5620 (59.309, 3.683) -> (58.801, 3.683)
  arc A3197 (59.3027, 6.223) -> (58.8073, 6.223) centre (59.055, 6.223) ccw
  arc A3198 (58.8073, 6.223) -> (59.3027, 6.223) centre (59.055, 6.223) ccw
  arc A3199 (59.055, 4.0767) -> (59.055, 3.2893) centre (59.055, 3.683) ccw
  line L5621 (59.309, 6.223) -> (58.801, 6.223)
  line L5622 (59.055, 6.477) -> (59.055, 5.969)
  arc A3200 (58.8073, 6.223) -> (59.3027, 6.223) centre (59.055, 6.223) ccw
  arc A3201 (58.8073, 6.223) -> (59.3027, 6.223) centre (59.055, 6.223) ccw
  line L5623 (59.309, 6.223) -> (58.801, 6.223)
  arc A3202 (59.055, 4.0767) -> (59.055, 3.2893) centre (59.055, 3.683) ccw
  arc A3203 (59.055, 3.2893) -> (59.055, 4.0767) centre (59.055, 3.683) ccw
  arc A3204 (59.3027, 6.223) -> (58.8073, 6.223) centre (59.055, 6.223) ccw
  line L5624 (59.309, 6.223) -> (58.801, 6.223)
  line L5625 (59.055, 6.477) -> (59.055, 5.969)
  arc A3205 (59.3027, 6.223) -> (58.8073, 6.223) centre (59.055, 6.223) ccw
  line L5626 (59.055, 6.477) -> (59.055, 5.969)
  line L5627 (59.055, 6.477) -> (59.055, 5.969)
  line L5628 (59.055, 3.937) -> (59.055, 3.429)
  arc A3206 (59.055, 6.6167) -> (59.055, 5.8293) centre (59.055, 6.223) ccw
  arc A3207 (59.055, 5.8293) -> (59.055, 6.6167) centre (59.055, 6.223) ccw
  arc A3208 (59.055, 3.2893) -> (59.055, 4.0767) centre (59.055, 3.683) ccw
  line L5629 (59.309, 6.223) -> (58.801, 6.223)
  line L5630 (61.849, 3.683) -> (61.341, 3.683)
  arc A3209 (61.8427, 6.223) -> (61.3473, 6.223) centre (61.595, 6.223) ccw
  arc A3210 (61.8427, 3.683) -> (61.3473, 3.683) centre (61.595, 3.683) ccw
  arc A3211 (61.595, 3.2893) -> (61.595, 4.0767) centre (61.595, 3.683) ccw
  arc A3212 (61.595, 5.8293) -> (61.595, 6.6167) centre (61.595, 6.223) ccw
  line L5631 (61.849, 6.223) -> (61.341, 6.223)
  arc A3213 (59.055, 6.6167) -> (59.055, 5.8293) centre (59.055, 6.223) ccw
  arc A3214 (61.8427, 3.683) -> (61.3473, 3.683) centre (61.595, 3.683) ccw
  line L5632 (61.849, 3.683) -> (61.341, 3.683)
  line L5633 (61.849, 6.223) -> (61.341, 6.223)
  arc A3215 (61.3473, 6.223) -> (61.8427, 6.223) centre (61.595, 6.223) ccw
  arc A3216 (61.3473, 3.683) -> (61.8427, 3.683) centre (61.595, 3.683) ccw
  line L5634 (61.849, 3.683) -> (61.341, 3.683)
  line L5635 (61.849, 3.683) -> (61.341, 3.683)
  arc A3217 (61.3473, 3.683) -> (61.8427, 3.683) centre (61.595, 3.683) ccw
  arc A3218 (59.055, 6.6167) -> (59.055, 5.8293) centre (59.055, 6.223) ccw
  line L5636 (61.595, 3.937) -> (61.595, 3.429)
  arc A3219 (61.3473, 3.683) -> (61.8427, 3.683) centre (61.595, 3.683) ccw
  line L5637 (61.595, 3.937) -> (61.595, 3.429)
  arc A3220 (61.8427, 3.683) -> (61.3473, 3.683) centre (61.595, 3.683) ccw
  arc A3221 (59.055, 5.969) -> (59.055, 6.477) centre (59.055, 6.223) ccw
  line L5638 (61.849, 3.683) -> (61.341, 3.683)
  arc A3222 (61.3473, 3.683) -> (61.8427, 3.683) centre (61.595, 3.683) ccw
  line L5639 (61.849, 3.683) -> (61.341, 3.683)
  arc A3223 (61.595, 3.2893) -> (61.595, 4.0767) centre (61.595, 3.683) ccw
  line L5640 (61.849, 3.683) -> (61.341, 3.683)
  line L5641 (61.595, 3.937) -> (61.595, 3.429)
  arc A3224 (59.055, 5.8293) -> (59.055, 6.6167) centre (59.055, 6.223) ccw
  arc A3225 (61.3473, 3.683) -> (61.8427, 3.683) centre (61.595, 3.683) ccw
  arc A3226 (61.595, 4.0767) -> (61.595, 3.2893) centre (61.595, 3.683) ccw
  arc A3227 (61.595, 4.0767) -> (61.595, 3.2893) centre (61.595, 3.683) ccw
  arc A3228 (61.595, 3.2893) -> (61.595, 4.0767) centre (61.595, 3.683) ccw
  arc A3229 (61.595, 3.2893) -> (61.595, 4.0767) centre (61.595, 3.683) ccw
  line L5642 (61.849, 6.223) -> (61.341, 6.223)
  arc A3230 (61.8427, 3.683) -> (61.3473, 3.683) centre (61.595, 3.683) ccw
  arc A3231 (61.3473, 3.683) -> (61.8427, 3.683) centre (61.595, 3.683) ccw
  line L5643 (61.595, 3.937) -> (61.595, 3.429)
  arc A3232 (61.595, 3.937) -> (61.595, 3.429) centre (61.595, 3.683) ccw
  arc A3233 (61.3473, 3.683) -> (61.8427, 3.683) centre (61.595, 3.683) ccw
  arc A3234 (59.055, 5.8293) -> (59.055, 6.6167) centre (59.055, 6.223) ccw
  arc A3235 (61.8427, 3.683) -> (61.3473, 3.683) centre (61.595, 3.683) ccw
  arc A3236 (61.3473, 3.683) -> (61.8427, 3.683) centre (61.595, 3.683) ccw
  line L5644 (61.595, 3.937) -> (61.595, 3.429)
  arc A3237 (59.055, 6.6167) -> (59.055, 5.8293) centre (59.055, 6.223) ccw
  line L5645 (61.595, 3.937) -> (61.595, 3.429)
  arc A3238 (61.8427, 3.683) -> (61.3473, 3.683) centre (61.595, 3.683) ccw
  line L5646 (61.849, 3.683) -> (61.341, 3.683)
  arc A3239 (61.3473, 3.683) -> (61.8427, 3.683) centre (61.595, 3.683) ccw
  line L5647 (61.595, 3.937) -> (61.595, 3.429)
  line L5648 (61.849, 3.683) -> (61.341, 3.683)
  arc A3240 (61.3473, 3.683) -> (61.8427, 3.683) centre (61.595, 3.683) ccw
  arc A3241 (61.8427, 3.683) -> (61.3473, 3.683) centre (61.595, 3.683) ccw
  arc A3242 (59.055, 5.8293) -> (59.055, 6.6167) centre (59.055, 6.223) ccw
  arc A3243 (59.055, 6.477) -> (59.055, 5.969) centre (59.055, 6.223) ccw
  arc A3244 (59.055, 6.6167) -> (59.055, 5.8293) centre (59.055, 6.223) ccw
  arc A3245 (61.595, 6.6167) -> (61.595, 5.8293) centre (61.595, 6.223) ccw
  arc A3246 (61.3473, 6.223) -> (61.8427, 6.223) centre (61.595, 6.223) ccw
  arc A3247 (61.8427, 6.223) -> (61.3473, 6.223) centre (61.595, 6.223) ccw
  line L5649 (61.595, 6.477) -> (61.595, 5.969)
  line L5650 (61.595, 6.477) -> (61.595, 5.969)
  line L5651 (61.849, 6.223) -> (61.341, 6.223)
  line L5652 (61.849, 6.223) -> (61.341, 6.223)
  arc A3248 (59.055, 5.8293) -> (59.055, 6.6167) centre (59.055, 6.223) ccw
  arc A3249 (61.8427, 6.223) -> (61.3473, 6.223) centre (61.595, 6.223) ccw
  line L5653 (64.389, 3.683) -> (63.881, 3.683)
  arc A3250 (64.3827, 3.683) -> (63.8873, 3.683) centre (64.135, 3.683) ccw
  arc A3251 (61.595, 3.2893) -> (61.595, 4.0767) centre (61.595, 3.683) ccw
  line L5654 (64.135, 3.937) -> (64.135, 3.429)
  arc A3252 (63.8873, 3.683) -> (64.3827, 3.683) centre (64.135, 3.683) ccw
  arc A3253 (64.135, 4.0767) -> (64.135, 3.2893) centre (64.135, 3.683) ccw
  arc A3254 (63.8873, 3.683) -> (64.3827, 3.683) centre (64.135, 3.683) ccw
  line L5655 (61.849, 6.223) -> (61.341, 6.223)
  arc A3255 (64.3827, 3.683) -> (63.8873, 3.683) centre (64.135, 3.683) ccw
  arc A3256 (64.135, 3.2893) -> (64.135, 4.0767) centre (64.135, 3.683) ccw
  arc A3257 (61.595, 3.429) -> (61.595, 3.937) centre (61.595, 3.683) ccw
  arc A3258 (61.3473, 6.223) -> (61.8427, 6.223) centre (61.595, 6.223) ccw
  arc A3259 (61.3473, 6.223) -> (61.8427, 6.223) centre (61.595, 6.223) ccw
  line L5656 (61.849, 6.223) -> (61.341, 6.223)
  arc A3260 (61.595, 5.8293) -> (61.595, 6.6167) centre (61.595, 6.223) ccw
  line L5657 (61.595, 6.477) -> (61.595, 5.969)
  arc A3261 (61.595, 6.6167) -> (61.595, 5.8293) centre (61.595, 6.223) ccw
  line L5658 (61.595, 6.477) -> (61.595, 5.969)
  line L5659 (64.389, 3.683) -> (63.881, 3.683)
  arc A3262 (61.3473, 6.223) -> (61.8427, 6.223) centre (61.595, 6.223) ccw
  arc A3263 (64.3827, 3.683) -> (63.8873, 3.683) centre (64.135, 3.683) ccw
  arc A3264 (61.8427, 6.223) -> (61.3473, 6.223) centre (61.595, 6.223) ccw
  arc A3265 (63.8873, 3.683) -> (64.3827, 3.683) centre (64.135, 3.683) ccw
  arc A3266 (64.3827, 3.683) -> (63.8873, 3.683) centre (64.135, 3.683) ccw
  line L5660 (64.389, 3.683) -> (63.881, 3.683)
  arc A3267 (63.8873, 3.683) -> (64.3827, 3.683) centre (64.135, 3.683) ccw
  arc A3268 (64.135, 3.2893) -> (64.135, 4.0767) centre (64.135, 3.683) ccw
  arc A3269 (61.595, 5.8293) -> (61.595, 6.6167) centre (61.595, 6.223) ccw
  line L5661 (64.135, 3.937) -> (64.135, 3.429)
  line L5662 (64.389, 3.683) -> (63.881, 3.683)
  line L5663 (64.135, 3.937) -> (64.135, 3.429)
  arc A3270 (61.595, 6.6167) -> (61.595, 5.8293) centre (61.595, 6.223) ccw
  arc A3271 (61.3473, 6.223) -> (61.8427, 6.223) centre (61.595, 6.223) ccw
  line L5664 (64.389, 3.683) -> (63.881, 3.683)
  arc A3272 (64.3827, 3.683) -> (63.8873, 3.683) centre (64.135, 3.683) ccw
  arc A3273 (61.3473, 6.223) -> (61.8427, 6.223) centre (61.595, 6.223) ccw
  arc A3274 (64.3827, 3.683) -> (63.8873, 3.683) centre (64.135, 3.683) ccw
  arc A3275 (61.595, 6.6167) -> (61.595, 5.8293) centre (61.595, 6.223) ccw
  arc A3276 (61.595, 6.477) -> (61.595, 5.969) centre (61.595, 6.223) ccw
  line L5665 (61.849, 6.223) -> (61.341, 6.223)
  line L5666 (61.595, 6.477) -> (61.595, 5.969)
  arc A3277 (61.3473, 6.223) -> (61.8427, 6.223) centre (61.595, 6.223) ccw
  line L5667 (61.595, 6.477) -> (61.595, 5.969)
  arc A3278 (61.595, 5.8293) -> (61.595, 6.6167) centre (61.595, 6.223) ccw
  arc A3279 (61.8427, 6.223) -> (61.3473, 6.223) centre (61.595, 6.223) ccw
  arc A3280 (61.595, 4.0767) -> (61.595, 3.2893) centre (61.595, 3.683) ccw
  arc A3281 (61.8427, 6.223) -> (61.3473, 6.223) centre (61.595, 6.223) ccw
  line L5668 (61.595, 6.477) -> (61.595, 5.969)
  arc A3282 (61.8427, 6.223) -> (61.3473, 6.223) centre (61.595, 6.223) ccw
  arc A3283 (61.8427, 6.223) -> (61.3473, 6.223) centre (61.595, 6.223) ccw
  line L5669 (61.595, 6.477) -> (61.595, 5.969)
  arc A3284 (61.595, 4.0767) -> (61.595, 3.2893) centre (61.595, 3.683) ccw
  line L5670 (61.595, 6.477) -> (61.595, 5.969)
  line L5671 (61.595, 6.477) -> (61.595, 5.969)
  arc A3285 (61.595, 5.969) -> (61.595, 6.477) centre (61.595, 6.223) ccw
  line L5672 (61.849, 6.223) -> (61.341, 6.223)
  arc A3286 (61.8427, 6.223) -> (61.3473, 6.223) centre (61.595, 6.223) ccw
  arc A3287 (61.8427, 6.223) -> (61.3473, 6.223) centre (61.595, 6.223) ccw
  arc A3288 (61.3473, 6.223) -> (61.8427, 6.223) centre (61.595, 6.223) ccw
  arc A3289 (64.135, 3.2893) -> (64.135, 4.0767) centre (64.135, 3.683) ccw
  arc A3290 (64.135, 4.0767) -> (64.135, 3.2893) centre (64.135, 3.683) ccw
  arc A3291 (64.135, 3.2893) -> (64.135, 4.0767) centre (64.135, 3.683) ccw
  line L5673 (61.849, 6.223) -> (61.341, 6.223)
  arc A3292 (61.3473, 6.223) -> (61.8427, 6.223) centre (61.595, 6.223) ccw
  arc A3293 (64.135, 5.8293) -> (64.135, 6.6167) centre (64.135, 6.223) ccw
  line L5674 (64.135, 6.477) -> (64.135, 5.969)
  line L5675 (64.135, 3.937) -> (64.135, 3.429)
  arc A3294 (64.3827, 6.223) -> (63.8873, 6.223) centre (64.135, 6.223) ccw
  line L5676 (64.135, 6.477) -> (64.135, 5.969)
  arc A3295 (61.595, 5.8293) -> (61.595, 6.6167) centre (61.595, 6.223) ccw
  line L5677 (64.135, 3.937) -> (64.135, 3.429)
  arc A3296 (64.135, 3.2893) -> (64.135, 4.0767) centre (64.135, 3.683) ccw
  arc A3297 (64.3827, 6.223) -> (63.8873, 6.223) centre (64.135, 6.223) ccw
  line L5678 (64.389, 6.223) -> (63.881, 6.223)
  line L5679 (50.165, 3.8608) -> (50.165, 6.8072)
  line L5680 (42.545, 3.8608) -> (50.165, 3.8608)
  arc A3298 (63.8873, 6.223) -> (64.3827, 6.223) centre (64.135, 6.223) ccw
  line L5681 (64.389, 6.223) -> (63.881, 6.223)
  arc A3299 (64.135, 3.937) -> (64.135, 3.429) centre (64.135, 3.683) ccw
  line L5682 (64.135, 3.937) -> (64.135, 3.429)
  line L5683 (64.389, 3.683) -> (63.881, 3.683)
  arc A3300 (63.8873, 3.683) -> (64.3827, 3.683) centre (64.135, 3.683) ccw
  arc A3301 (64.3827, 3.683) -> (63.8873, 3.683) centre (64.135, 3.683) ccw
  arc A3302 (64.135, 3.429) -> (64.135, 3.937) centre (64.135, 3.683) ccw
  arc A3303 (64.135, 6.6167) -> (64.135, 5.8293) centre (64.135, 6.223) ccw
  arc A3304 (63.8873, 3.683) -> (64.3827, 3.683) centre (64.135, 3.683) ccw
  arc A3305 (61.595, 6.6167) -> (61.595, 5.8293) centre (61.595, 6.223) ccw
  line L5684 (64.389, 3.683) -> (63.881, 3.683)
  arc A3306 (64.3827, 6.223) -> (63.8873, 6.223) centre (64.135, 6.223) ccw
  arc A3307 (64.135, 4.0767) -> (64.135, 3.2893) centre (64.135, 3.683) ccw
  arc A3308 (64.135, 5.969) -> (64.135, 6.477) centre (64.135, 6.223) ccw
  line L5685 (64.135, 6.477) -> (64.135, 5.969)
  line L5686 (64.135, 3.937) -> (64.135, 3.429)
  arc A3309 (64.3827, 6.223) -> (63.8873, 6.223) centre (64.135, 6.223) ccw
  arc A3310 (64.135, 6.6167) -> (64.135, 5.8293) centre (64.135, 6.223) ccw
  line L5687 (42.545, 6.8072) -> (42.545, 3.8608)
  line L5688 (64.389, 6.223) -> (63.881, 6.223)
  arc A3311 (64.135, 5.8293) -> (64.135, 6.6167) centre (64.135, 6.223) ccw
  arc A3312 (64.135, 6.6167) -> (64.135, 5.8293) centre (64.135, 6.223) ccw
  line L5689 (64.135, 3.937) -> (64.135, 3.429)
  line L5690 (64.135, 3.937) -> (64.135, 3.429)
  arc A3313 (64.135, 4.0767) -> (64.135, 3.2893) centre (64.135, 3.683) ccw
  line L5691 (64.135, 3.937) -> (64.135, 3.429)
  line L5692 (64.389, 3.683) -> (63.881, 3.683)
  arc A3314 (63.8873, 3.683) -> (64.3827, 3.683) centre (64.135, 3.683) ccw
  arc A3315 (64.3827, 3.683) -> (63.8873, 3.683) centre (64.135, 3.683) ccw
  line L5693 (64.389, 3.683) -> (63.881, 3.683)
  arc A3316 (64.3827, 3.683) -> (63.8873, 3.683) centre (64.135, 3.683) ccw
  line L5694 (64.389, 3.683) -> (63.881, 3.683)
  arc A3317 (63.8873, 3.683) -> (64.3827, 3.683) centre (64.135, 3.683) ccw
  arc A3318 (64.3827, 3.683) -> (63.8873, 3.683) centre (64.135, 3.683) ccw
  arc A3319 (64.135, 4.0767) -> (64.135, 3.2893) centre (64.135, 3.683) ccw
  arc A3320 (63.8873, 6.223) -> (64.3827, 6.223) centre (64.135, 6.223) ccw
  arc A3321 (63.8873, 3.683) -> (64.3827, 3.683) centre (64.135, 3.683) ccw
  arc A3322 (64.3827, 6.223) -> (63.8873, 6.223) centre (64.135, 6.223) ccw
  arc A3323 (64.135, 5.8293) -> (64.135, 6.6167) centre (64.135, 6.223) ccw
  arc A3324 (63.8873, 3.683) -> (64.3827, 3.683) centre (64.135, 3.683) ccw
  line L5695 (64.135, 6.477) -> (64.135, 5.969)
  arc A3325 (63.8873, 6.223) -> (64.3827, 6.223) centre (64.135, 6.223) ccw
  arc A3326 (64.135, 5.8293) -> (64.135, 6.6167) centre (64.135, 6.223) ccw
  line L5696 (64.135, 6.477) -> (64.135, 5.969)
  arc A3327 (64.135, 6.6167) -> (64.135, 5.8293) centre (64.135, 6.223) ccw
  arc A3328 (63.8873, 6.223) -> (64.3827, 6.223) centre (64.135, 6.223) ccw
  line L5697 (50.165, 6.8072) -> (42.545, 6.8072)
  arc A3329 (63.8873, 6.223) -> (64.3827, 6.223) centre (64.135, 6.223) ccw
  line L5698 (64.135, 6.477) -> (64.135, 5.969)
  arc A3330 (64.135, 6.6167) -> (64.135, 5.8293) centre (64.135, 6.223) ccw
  line L5699 (64.389, 6.223) -> (63.881, 6.223)
  arc A3331 (43.815, 4.9403) -> (43.815, 5.7277) centre (43.815, 5.334) ccw
  arc A3332 (43.815, 5.7277) -> (43.815, 4.9403) centre (43.815, 5.334) ccw
  arc A3333 (63.8873, 6.223) -> (64.3827, 6.223) centre (64.135, 6.223) ccw
  arc A3334 (43.815, 5.08) -> (43.815, 5.588) centre (43.815, 5.334) ccw
  line L5700 (43.561, 5.334) -> (44.069, 5.334)
  arc A3335 (43.5673, 5.334) -> (44.0627, 5.334) centre (43.815, 5.334) ccw
  arc A3336 (44.0627, 5.334) -> (43.5673, 5.334) centre (43.815, 5.334) ccw
  line L5701 (64.389, 6.223) -> (63.881, 6.223)
  line L5702 (43.815, 5.08) -> (43.815, 5.588)
  line L5703 (50.8, 6.8072) -> (41.91, 6.8072)
  arc A3337 (43.5673, 5.334) -> (44.0627, 5.334) centre (43.815, 5.334) ccw
  arc A3338 (64.135, 5.8293) -> (64.135, 6.6167) centre (64.135, 6.223) ccw
  arc A3339 (64.3827, 6.223) -> (63.8873, 6.223) centre (64.135, 6.223) ccw
  line L5704 (64.389, 6.223) -> (63.881, 6.223)
  arc A3340 (44.0627, 5.334) -> (43.5673, 5.334) centre (43.815, 5.334) ccw
  arc A3341 (43.815, 5.588) -> (43.815, 5.08) centre (43.815, 5.334) ccw
  line L5705 (64.135, 6.477) -> (64.135, 5.969)
  line L5706 (43.561, 5.334) -> (44.069, 5.334)
  line L5707 (43.561, 5.334) -> (44.069, 5.334)
  line L5708 (64.389, 6.223) -> (63.881, 6.223)
  line L5709 (43.561, 5.334) -> (44.069, 5.334)
  line L5710 (43.0276, 5.334) -> (44.6024, 5.334)
  line L5711 (43.561, 5.334) -> (44.069, 5.334)
  arc A3342 (43.5673, 5.334) -> (44.0627, 5.334) centre (43.815, 5.334) ccw
  arc A3343 (44.0627, 5.334) -> (43.5673, 5.334) centre (43.815, 5.334) ccw
  line L5712 (43.815, 5.08) -> (43.815, 5.588)
  line L5713 (43.561, 5.334) -> (44.069, 5.334)
  arc A3344 (43.5673, 5.334) -> (44.0627, 5.334) centre (43.815, 5.334) ccw
  arc A3345 (43.5673, 5.334) -> (44.0627, 5.334) centre (43.815, 5.334) ccw
  line L5714 (43.0276, 5.334) -> (44.6024, 5.334)
  line L5715 (43.0276, 5.334) -> (44.6024, 5.334)
  arc A3346 (64.3827, 6.223) -> (63.8873, 6.223) centre (64.135, 6.223) ccw
  arc A3347 (64.3827, 6.223) -> (63.8873, 6.223) centre (64.135, 6.223) ccw
  arc A3348 (43.5673, 5.334) -> (44.0627, 5.334) centre (43.815, 5.334) ccw
  arc A3349 (44.0627, 5.334) -> (43.5673, 5.334) centre (43.815, 5.334) ccw
  line L5716 (43.561, 5.334) -> (44.069, 5.334)
  arc A3350 (44.0627, 5.334) -> (43.5673, 5.334) centre (43.815, 5.334) ccw
  line L5717 (64.389, 6.223) -> (63.881, 6.223)
  arc A3351 (63.8873, 6.223) -> (64.3827, 6.223) centre (64.135, 6.223) ccw
  arc A3352 (63.8873, 6.223) -> (64.3827, 6.223) centre (64.135, 6.223) ccw
  line L5718 (64.135, 6.477) -> (64.135, 5.969)